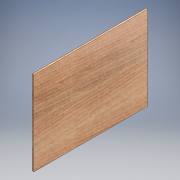
# Autodesk Inventor part: cloison_porte-monnayeur
Saved by Autodesk Inventor 2018 (Build 220112000, 112)
## iProperties
Created: 2018-12-03
Part Number: cloison_porte-monnayeur
Material: Wood (Birch)
Document SubType Name: Modeling
Designer: Bienvenue
Density: 0.55 g/cm^3
Appearance: Birch - Natural Polished
Author: Bienvenue
Autodesk Inventor part; units mm, degrees
ref_plane "YZ Plane" through (0, 0, 0) normal (1, 0, 0) x (0, 1, 0)
ref_plane "XZ Plane" through (0, 0, 0) normal (0, 1, 0) x (-1, 0, 0)
ref_plane "XY Plane" through (0, 0, 0) normal (0, 0, 1) x (1, 0, 0)
sketch "Sketch1" plane through (0, 0, 0) normal (1, 0, 0) x (0, 1, 0)
  line L0 (0, 0) -> (400, 0)
  line L1 (400, 0) -> (400, -300)
  line L2 (400, -300) -> (0, -300)
  line L3 (0, -300) -> (0, 0)
  dimension "d0" = 400
  dimension "d1" = 300
  constraints: 8 end point, 2 parallel, 1 horizontal, 1 perpendicular
  measures "d0" distance of L1.end L2.end
  measures "d1" distance of L0.end L1.end
extrude "Extrusion1" add sketch "Sketch1" along normal blind 6
sketch "Sketch2" plane through (6, 0, 0) normal (1, 0, 0) x (0, 0, -1)
  line L0 (0, 0) -> (299.9643, 0)
  line L1 (299.9643, 0) -> (299.9643, -6)
  line L2 (299.9643, -6) -> (0, -6)
  line L3 (0, -6) -> (0, 0)
  dimension "d4" = 6
  constraints: 8 end point, 2 parallel, 1 horizontal, 1 perpendicular
  measures "d4" distance of L2.end L0.start
extrude "Extrusion2" add sketch "Sketch2" against normal blind 6
body "Solid1"
